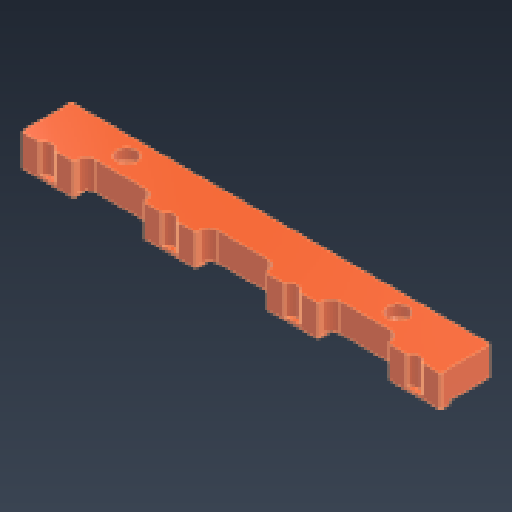
# Autodesk Inventor part: VEJ-00-112
Saved by Autodesk Inventor 2026.1 (Build 301233000, 233)
## iProperties
Created: 2025-08-16
Part Number: VEJ-00-112
Material: Fenolite OR
Document SubType Name: Modeling
Designer: Willian Pinheiro
Mass: 22.8662 g
Surface Area: 69.6673 cm^2
Volume: 16.5697 cm^3
Density: 1.38 g/cm^3
Appearance: Suave - Laranja claro
Description: Suporte LED PCB 17117000005183-1.3
Project: VEJ-00
Checked By: Antonio Lucas
Engr Approved By: Antonio Lucas
Mfg Approved By: Anderson Oliveira
Company: Venttos
Dimensões: 10 x 16 x 133 mm
Total: 1
Author: Willian Pinheiro
Revision Number: 00
Title: Palete
Autodesk Inventor part; units mm, degrees
ref_plane "YZ Plane" through (0, 0, 0) normal (1, 0, 0) x (0, 1, 0)
ref_plane "XZ Plane" through (0, 0, 0) normal (0, 1, 0) x (-1, 0, 0)
ref_plane "XY Plane" through (0, 0, 0) normal (0, 0, 1) x (1, 0, 0)
sketch "Esboço1" plane through (0, 0, 0) normal (0, 0, 1) x (1, 0, 0)
  line L0 (-124.04, 0) -> (124.04, 0) construction
  line L1 (0, -17.8) -> (0, 12.3) construction
  line L2 (-74.5, 8) -> (74.5, 8)
  line L3 (74.5, 8) -> (74.5, -8)
  line L4 (74.5, -8) -> (-74.5, -8)
  line L5 (-74.5, -8) -> (-74.5, 8)
  line L6 (-74.5, 2) -> (74.5, 2) construction
  line L7 (-49.8, -8) -> (-27.8, -8)
  line L8 (-27.8, -8) -> (-27.8, -4)
  line L9 (-27.8, -4) -> (-49.8, -4)
  line L10 (-49.8, -4) -> (-49.8, -8)
  line L11 (49.8, -8) -> (27.8, -8)
  line L12 (27.8, -8) -> (27.8, -4)
  line L13 (27.8, -4) -> (49.8, -4)
  line L14 (49.8, -4) -> (49.8, -8)
  line L15 (-19.4, -8) -> (-19.4, 8) construction
  line L16 (11, -8) -> (-11, -8)
  line L17 (-11, -8) -> (-11, -4)
  line L18 (-11, -4) -> (11, -4)
  line L19 (11, -4) -> (11, -8)
  line L20 (-58.2, -8) -> (-58.2, 8) construction
  line L21 (-38.8, -4) -> (-38.8, -8) construction
  line L22 (-66.6, -8) -> (-88.6, -8)
  line L23 (-88.6, -8) -> (-88.6, -4)
  line L24 (-88.6, -4) -> (-66.6, -4)
  line L25 (-66.6, -4) -> (-66.6, -8)
  line L26 (-77.6, -4) -> (-77.6, -8) construction
  line L27 (88.6, -8) -> (88.6, -4)
  line L28 (77.6, -4) -> (77.6, -8) construction
  line L29 (88.6, -4) -> (66.6, -4)
  line L30 (66.6, -8) -> (88.6, -8)
  line L31 (66.6, -4) -> (66.6, -8)
  line L32 (-66.5, 8) -> (-66.5, -8)
  line L33 (66.5, 8) -> (66.5, -8)
  line L34 (-74.5, -6) -> (74.5, -6)
  line L35 (-19.4, -11) -> (-19.4, -9) construction
  line L36 (-16.9, -11) -> (-16.9, -9)
  line L37 (-21.9, -9) -> (-21.9, -11)
  arc A0 (-21.9, -11) -> (-16.9, -11) centre (-19.4, -11) ccw
  arc A1 (-16.9, -9) -> (-21.9, -9) centre (-19.4, -9) ccw
  line L38 (-58.2, -11) -> (-58.2, -9) construction
  line L39 (-60.7, -11) -> (-60.7, -9)
  line L40 (-55.7, -9) -> (-55.7, -11)
  arc A2 (-60.7, -11) -> (-55.7, -11) centre (-58.2, -11) ccw
  arc A3 (-55.7, -9) -> (-60.7, -9) centre (-58.2, -9) ccw
  line L41 (19.4, -11) -> (19.4, -9) construction
  line L42 (16.9, -11) -> (16.9, -9)
  line L43 (21.9, -9) -> (21.9, -11)
  arc A4 (16.9, -11) -> (21.9, -11) centre (19.4, -11) ccw
  arc A5 (21.9, -9) -> (16.9, -9) centre (19.4, -9) ccw
  arc A6 (60.7, -9) -> (55.7, -9) centre (58.2, -9) ccw
  line L44 (55.7, -9) -> (55.7, -11)
  line L45 (58.2, -11) -> (58.2, -9) construction
  line L46 (60.7, -11) -> (60.7, -9)
  arc A7 (55.7, -11) -> (60.7, -11) centre (58.2, -11) ccw
  line L47 (74.5, -4.5) -> (-74.5, -4.5)
  line L48 (-74.5, -4.5) -> (-74.5, 8)
  line L49 (-74.5, 8) -> (74.5, 8)
  line L50 (74.5, 8) -> (74.5, -4.5)
  point P0 (0, 0)
  point P1 (-43, 2)
  point P2 (43, 2)
  point P3 (0, -4)
  point P4 (66.5, -6)
  point P5 (49.8, -6)
  point P6 (-66.5, -6)
  point P7 (-19.4, -10)
  point P8 (-58.2, -10)
  point P9 (19.4, -8)
  point P10 (58.2, -8)
  point P11 (19.4, -10)
  point P12 (58.2, -10)
  point P13 (11, -4)
  point P14 (-74.5, -4)
  point P15 (-11, -4.5)
  point P16 (11, -4.5)
  point P17 (27.8, -4.5)
  point P18 (49.8, -4.5)
  point P19 (-27.8, -4.5)
  point P20 (66.6, -4.5)
  point P21 (74.5, -4)
  point P22 (-66.6, -4.5)
  point P23 (-49.8, -4.5)
  dimension "d0" = 149
  dimension "d1" = 16
  dimension "d2" = 6
  dimension "d4" = 86
  dimension "d5" = 4
  dimension "d6" = 22
  dimension "d7" = 38.8
  dimension "d8" = 133
  dimension "d9" = 23.5
  dimension "d12" = 2
  dimension "d23" = 5
  dimension "d24" = 1.5
  dimension "d25" = 2
  dimension "d36" = 12.5
  constraints: 106 end point, 46 symmetric about line, 16 point on circle, 14 point on line, 8 centre point, 7 parallel, 5 perpendicular, 4 horizontal, 4 midpoint, 4 tangent, 2 vertical, 1 collinear, 10 other
  measures "d0" distance of L2.start L2.end
  measures "d1" distance between parallel lines of L4 L2
  measures "d2" distance between parallel lines of L6 L2
  measures "d4" distance of point (43, 2) point (-43, 2)
  measures "d5" distance between parallel lines of L4 L9
  measures "d6" distance of L8.end L9.end
  measures "d7" distance of point (0, -4) L21.start
  measures "d8" distance between parallel lines of L33 L32
  measures "d9" distance from line of point (-43, 2) L32
  measures "d12" distance between parallel lines of L4 L34
  measures "d23" distance between parallel lines of L36 L37
  measures "d24" distance edge to line of A1 L4
  measures "d25" distance of L35.start L35.end
  measures "d36" distance between parallel lines of L2 L47
extrude "Extrusão1" add sketch "Esboço1" against normal blind 10 contours L2 L33 L47 L14 L13 L12 L19 L18 L17 L8 L9 L10 L32 | L47 L10 L34 L32 | L33 L34 L14 L47 | L34 L10 L4 A3 L32 | L33 L4 A6 L14 L34 | L47 L17 L34 L8 | L12 L34 L19 L47 | A3 L4 | L34 L17 L4 A1 L8 | L4 A6 | L12 L4 A5 L19 L34 | A1 L4 | L4 A5
extrude "Extrusão2" cut sketch "Esboço1" along normal blind 1 from surface at -10 contours L2 L32 L47 L25 L24 L5 | L2 L33 L47 L14 L13 L12 L19 L18 L17 L8 L9 L10 L32 | L24 L25 L47 L5 | L5 L22 L23 L24 | L2 L3 L29 L31 L47 L33
extrude "Extrusão3" cut sketch "Esboço1" against normal blind 8.5 contours A3 L4 | L4 A3 L40 A2 L39 | A6 L46 A7 L44 L4 | L4 A6 | A1 L4 | L4 A1 L36 A0 L37 | A5 L43 A4 L42 L4 | L4 A5
hole "Furo1" at (-43, 2, 0) at (43, 2, 0) direction (0, 0, -1) diameter 3.5 end through all counterbore diameter 6.5 counterbore depth 3.5 clearance for "Socket Head Cap Screw ISO 4762" size "M3" standard "ISO"
fillet "Arredondamento1" radius 0.5 26 edges at (66.5, -8, -5) (66.5, 8, -4.5) (-66.5, -8, -5) (-66.5, 8, -4.5) (-49.8, -8, -5) (-27.8, -8, -5) (-11, -8, -5) (11, -8, -5) (27.8, -8, -5) (49.8, -8, -5) (55.9087, -8, -4.25) (60.4913, -8, -4.25) (17.1087, -8, -4.25) (21.6913, -8, -4.25) (-21.6913, -8, -4.25) (-17.1087, -8, -4.25) (-60.4913, -8, -4.25) (-55.9087, -8, -4.25) (49.8, -4.5, -9.5) (27.8, -4.5, -9.5) (11, -4.5, -9.5) (-11, -4.5, -9.5) (-27.8, -4.5, -9.5) (-49.8, -4.5, -9.5) (-66.5, -4.5, -9.5) (66.5, -4.5, -9.5)
fillet "Arredondamento1" radius 3 6 edges at (-49.8, -4, -4.5) (-27.8, -4, -4.5) (-11, -4, -4.5) (11, -4, -4.5) (27.8, -4, -4.5) (49.8, -4, -4.5)
chamfer "Chanfro1" distance 1.5 angle 45 2 edges at (-43, 3.75, -3.5) (43, 3.75, -3.5)
